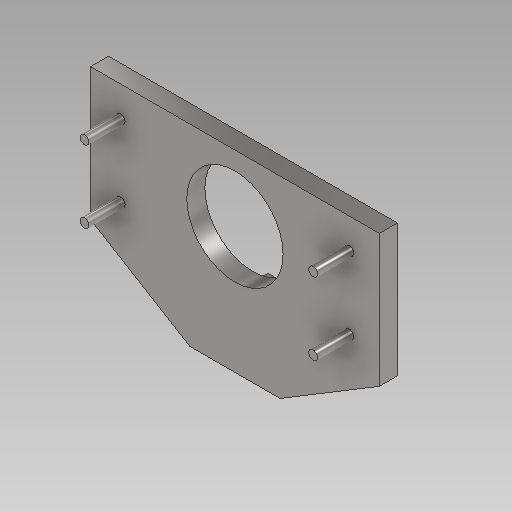
# Autodesk Inventor part: soporte
Saved by Autodesk Inventor 2021 (Build 250183000, 183)
## iProperties
Created: 2022-01-31
Part Number: soporte
Material: Acerito
Document SubType Name: Modeling
Designer: Osmar Ediber Toloza Bernal
Density: 8 g/cm^3
Appearance: Semipulido
Mass: 33634.1 g
Surface Area: 3524.48 cm^2
Volume: 4204.26 cm^3
Author: Osmar Ediber Toloza Bernal
Autodesk Inventor part; units mm, degrees
ref_plane "YZ Plane" through (0, 0, 0) normal (1, 0, 0) x (0, 1, 0)
ref_plane "XZ Plane" through (0, 0, 0) normal (0, 1, 0) x (-1, 0, 0)
sketch "Boceto1" plane through (0, 0, 0) normal (0, 0, 1) x (1, 0, 0)
  circle A0 centre (0, 0) radius 264 construction
  line L0 (-239.9917, 110) -> (239.9917, 110)
  line L1 (239.9917, 110) -> (239.9917, -110)
  line L2 (239.9917, -110) -> (-239.9917, -110)
  line L3 (-239.9917, -110) -> (-239.9917, 110)
  line L4 (-239.9917, 110) -> (239.9917, -110) construction
  line L5 (239.9917, 110) -> (-239.9917, -110) construction
  dimension "d0" = 528
  dimension "d1" = 220
  constraints: 12 end point, 2 coincident, 2 parallel, 2 point on circle, 1 centre point, 1 horizontal, 1 midpoint, 1 perpendicular
  measures "d0" diameter of A0
  measures "d1" distance of L0.end L1.end
extrude "Extrusión1" add sketch "Boceto1" along normal blind 30
sketch "Boceto2" plane through (0, 0, 30) normal (0, 0, 1) x (1, 0, 0)
  circle A0 centre (-189.9917, 60) radius 7.5
  line L0 (239.9917, 110) -> (-239.9917, 110) construction
  line L1 (-239.9917, 110) -> (-239.9917, -110) construction
  point P0 (0, 0)
  dimension "d4" = 15
  dimension "d5" = 50
  dimension "d6" = 50
  constraints: 1 centre point
  measures "d4" diameter of A0
  measures "d5" distance from line of L0 A0.centre
  measures "d6" distance from line of L1 A0.centre
extrude "Extrusión2" add sketch "Boceto2" along normal blind 60
mirror "Simetría1" about plane through (0, 0, 0) normal (1, 0, 0) of "Extrusión2"
mirror "Simetría2" about plane through (0, 0, 0) normal (0, 1, 0) of "Extrusión2", "Simetría1"
sketch "Boceto3" plane through (0, 0, 30) normal (0, 0, 1) x (1, 0, 0)
  circle A0 centre (0, 0) radius 80
  dimension "d17" = 160
  constraints: 1 centre point, 1 coincident
  measures "d17" diameter of A0
extrude "Extrusión3" cut sketch "Boceto3" along normal through all both and the other way through all
sketch "Boceto9" plane through (-239.9917, -110, 0) normal (0, -1, 0) x (1, 0, 0)
  line L0 (0, 30) -> (479.9833, 30) projected
  line L1 (479.9833, 0) -> (0, 0) projected
  line L2 (0, 30) -> (479.9833, 30)
  line L3 (479.9833, 30) -> (479.9833, 0)
  line L4 (479.9833, 0) -> (0, 0)
  line L5 (0, 0) -> (0, 30)
  point P0 (239.9917, 0)
  constraints: 8 end point, 2 parallel, 1 horizontal, 1 perpendicular
ref_plane "Plano de trabajo1" through (-239.9917, -210, 0) normal (0, -1, 0) x (1, 0, 0)
sketch "Boceto10" plane through (-239.9917, -210, 0) normal (0, -1, 0) x (1, 0, 0)
  line L0 (0, 0) -> (479.9833, 0) construction
  line L1 (479.9833, 0) -> (479.9833, 30) construction
  line L2 (0, 30) -> (479.9833, 30) construction
  line L3 (0, 0) -> (0, 30) construction
  line L4 (164.9917, 30) -> (314.9917, 30)
  line L5 (314.9917, 30) -> (314.9917, 0)
  line L6 (314.9917, 0) -> (164.9917, 0)
  line L7 (164.9917, 0) -> (164.9917, 30)
  point P0 (239.9917, 0)
  point P1 (239.9917, 30)
  dimension "d41" = 150
  dimension "d42" = 30
  constraints: 8 end point, 2 midpoint, 2 parallel, 1 horizontal, 1 perpendicular
  measures "d41" distance of L4.start L4.end
  measures "d42" distance of L4.end L5.end
loft "Solevación1" add profiles "Boceto10" section 1 edges at (0, -110, 0) (239.9917, -110, 15) (0, -110, 30) (-239.9917, -110, 15)
sketch "Boceto11" plane through (0, 0, 0) normal (0, 0, -1) x (-1, 0, 0)
  line L0 (75, -210) -> (-75, -210)
  line L1 (-75, -210) -> (-75, -170)
  line L2 (-75, -170) -> (75, -170)
  line L3 (75, -170) -> (75, -210)
  line L4 (-75, -210) -> (75, -210) projected
  point P0 (0, 0)
  point P1 (0, -210)
  dimension "d48" = 150
  dimension "d49" = 40
  constraints: 8 end point, 2 midpoint, 2 parallel, 1 horizontal, 1 perpendicular
  measures "d48" distance of L0.start L0.end
  measures "d49" distance of L0.end L1.end
extrude "Extrusión8" add sketch "Boceto11" along normal blind 100
sketch "Boceto12" plane through (-75, -210, 30) normal (0, -1, 0) x (1, 0, 0)
  line L0 (150, -130) -> (0, -130) construction
  line L1 (0, -30) -> (0, 0) construction
  line L2 (150, -130) -> (0, -130) construction
  line L3 (0, -130) -> (0, -30) construction
  line L4 (0, -30) -> (150, -30) construction
  line L5 (150, -30) -> (150, -130) construction
  line L6 (150, 0) -> (150, -30) construction
  line L7 (150, -30) -> (0, -130) construction
  line L8 (0, -30) -> (150, -130) construction
  circle A0 centre (75, -80) radius 31.5
  point P0 (75, -30)
  dimension "d52" = 63
  constraints: 12 end point, 2 parallel, 1 centre point, 1 horizontal, 1 midpoint, 1 perpendicular
  measures "d52" diameter of A0
extrude "Extrusión9" add sketch "Boceto12" along normal blind 20
sketch "Boceto13" plane through (0, -230, -50) normal (0, -1, 0) x (1, 0, 0)
  circle A0 centre (0, 0) radius 25 construction
  circle A1 centre (0, 25) radius 3
  circle A2 centre (0, -25) radius 3
  circle A3 centre (23.7764, -7.7254) radius 3
  circle A4 centre (14.6946, 20.2254) radius 3
  circle A5 centre (-14.6946, 20.2254) radius 3
  circle A6 centre (-23.7764, -7.7254) radius 3
  point P0 (0, 50)
  dimension "d55" = 50
  dimension "d56" = 6
  dimension "d57" = 6
  dimension "d60" = 360
  constraints: 7 centre point, 2 point on circle, 11 other
  measures "d55" diameter of A0
  measures "d56" diameter of A1
  measures "d57" diameter of A2
extrude "Extrusión10" cut sketch "Boceto13" against normal up to next
equation "\"d0\" = 0.8 * diametro_llanta"
equation "\"d1\" = 0.333333 * diametro_llanta"
equation "\"d2\" = espesor_soporte"
equation "\"d4\" = 0.5 * espesor_soporte"
equation "\"d7\" = 2 * espesor_soporte"
equation "\"d42\" = espesor_soporte"
equation "\"ancho_llanta\" = 271000"
equation "\"espesor_soporte\" = 30"
equation "\"diametro_llanta\" = 660"
